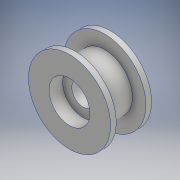
# Autodesk Inventor part: Idler Pulley
Saved by Autodesk Inventor 2017.3 (Build 213256000, 256)
## iProperties
Created: 2018-10-13
Part Number: Idler Pulley
Material: Aluminum 6061
Document SubType Name: Modeling
Designer: Ax
Density: 2.7 g/cm^3
Appearance: Aluminum - Flat
Author: Ax
Autodesk Inventor part; units mm, degrees
ref_plane "YZ Plane" through (0, 0, 0) normal (1, 0, 0) x (0, 1, 0)
ref_plane "XZ Plane" through (0, 0, 0) normal (0, 1, 0) x (-1, 0, 0)
ref_plane "XY Plane" through (0, 0, 0) normal (0, 0, 1) x (1, 0, 0)
sketch "Sketch1" plane through (0, 0, 0) normal (0, 0, 1) x (1, 0, 0)
  line L0 (0, 0) -> (2.5, 0) construction
  line L1 (2.5, 4.5) -> (2.5, -4.5)
  line L2 (2.5, -4.5) -> (9, -4.5)
  line L3 (9, -4.5) -> (9, -3.25)
  line L4 (9, -3.25) -> (6.05, -3.25)
  line L5 (6.05, -3.25) -> (6.05, 3.25)
  line L6 (6.05, 3.25) -> (9, 3.25)
  line L7 (9, 3.25) -> (9, 4.5)
  line L8 (9, 4.5) -> (2.5, 4.5)
  line L9 (0, -6.3) -> (0, 6.3) projected
  dimension "d0" = 2.5
  dimension "d1" = 6.5
  dimension "d2" = 9
  dimension "d3" = 9
  dimension "d4" = 6.05
  constraints: 18 end point, 7 perpendicular, 2 symmetric about line, 1 collinear, 1 midpoint, 1 vertical
  measures "d0" distance of L0.start L0.end
  measures "d1" distance of L4.end L5.end
  measures "d2" distance of L1.start L1.end
  measures "d3" horizontal distance of L0.start L7.end
  measures "d4" horizontal distance of L0.start L5.end
revolve "Revolution1" add sketch "Sketch1" angle 360 about axis through (0, -10, 0) along (0, 1, 0)
sketch "Sketch2" plane through (0, 4.5, 0) normal (0, 1, 0) x (1, 0, 0)
  circle A0 centre (0, 0) radius 4.5
  dimension "d6" = 9
  constraints: 1 centre point, 1 coincident
  measures "d6" diameter of A0
extrude "Extrusion1" cut sketch "Sketch2" against normal blind 3
mirror "Mirror1" about plane through (0, 0, 0) normal (0, 1, 0) of "Extrusion1"
body "Solid1"
